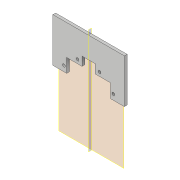
# Autodesk Inventor part: Hang Mount
Saved by Autodesk Inventor 2018 (Build 220112000, 112)
## iProperties
Created: 2018-01-17
Part Number: Hang Mount
Material: Generic
Document SubType Name: Modeling
Designer: dsayers
Density: 1 g/cm^3
Appearance: Default
Author: dsayers
Autodesk Inventor part; units mm, degrees
ref_plane "YZ Plane" through (0, 0, 0) normal (1, 0, 0) x (0, 1, 0)
ref_plane "XZ Plane" through (0, 0, 0) normal (0, 1, 0) x (-1, 0, 0)
ref_plane "XY Plane" through (0, 0, 0) normal (0, 0, 1) x (1, 0, 0)
ref_plane "Work Plane1" through (0, 0, 0) normal (0, 0, 1) x (1, 0, 0)
sketch "Sketch2" plane through (0, 0, 0) normal (0, 0, 1) x (1, 0, 0)
  line L0 (-69.85, 121.9708) -> (69.85, 121.9708) projected
  line L1 (-69.85, 33.0708) -> (-69.85, 121.9708) projected
  line L2 (69.85, 33.0708) -> (-69.85, 33.0708) projected
  line L3 (-50.8, 64.8208) -> (-50.8, 33.0708) projected
  line L4 (50.8, 64.8208) -> (-50.8, 64.8208) projected
  line L5 (50.8, 33.0708) -> (50.8, 64.8208) projected
  line L6 (69.85, 121.9708) -> (69.85, 33.0708) projected
  line L7 (-15.2718, 85.3756) -> (-15.2718, 64.8208) projected
  line L8 (15.24, 85.3756) -> (-15.2718, 85.3756) projected
  line L9 (15.24, 64.8208) -> (15.24, 85.3756) projected
  point P0 (0, 0)
extrude "Extrusion1" add sketch "Sketch2" along normal blind 6.35 contours L0 L6 L2 L5 L4 L9 L8 L7 L3 L1
sketch "Sketch3" plane through (0, 0, 6.35) normal (0, 0, 1) x (1, 0, 0)
  circle A0 centre (-57.15, 45.7708) radius 3.5662 projected
  circle A1 centre (-25.4, 73.7616) radius 2.4892 projected
  circle A2 centre (57.15, 45.7708) radius 3.9624 projected
  point P0 (0, 0)
  point P1 (25.4, 73.7616)
  point P2 (25.4, 73.7616)
  constraints: 4 coincident
hole "Hole1" at (25.4, 73.7616, 6.35) at (-57.15, 45.7708, 6.35) at (57.15, 45.7708, 6.35) at (-25.4, 73.7616, 6.35) direction (0, 0, -1) diameter 6.35 depth 25.4 tip angle 118
sketch "Sketch5" plane through (0, 0, 6.35) normal (0, 0, 1) x (1, 0, 0)
  line L0 (-69.85, 33.0708) -> (-50.8, 33.0708) projected
  line L1 (-69.85, 33.0708) -> (-82.55, 33.0708)
  line L2 (-82.55, 33.0708) -> (-82.55, 134.6708)
  line L3 (-82.55, 134.6708) -> (-69.85, 134.6708)
  line L4 (-69.85, 134.6708) -> (-69.85, 33.0708)
  line L5 (-82.55, 134.6708) -> (82.55, 134.6708)
  line L6 (82.55, 134.6708) -> (82.55, 121.9708)
  line L7 (82.55, 121.9708) -> (-82.55, 121.9708)
  line L8 (-82.55, 121.9708) -> (-82.55, 134.6708)
  line L9 (50.8, 33.0708) -> (69.85, 33.0708) projected
  line L10 (82.55, 121.9708) -> (69.85, 121.9708)
  line L11 (69.85, 121.9708) -> (69.85, 33.0708)
  line L12 (69.85, 33.0708) -> (82.55, 33.0708)
  line L13 (82.55, 33.0708) -> (82.55, 121.9708)
  point P0 (0, 0)
  dimension "d26" = 12.7
  dimension "d27" = 12.7
  dimension "d28" = 12.7
  constraints: 24 end point, 6 parallel, 3 horizontal, 3 perpendicular
  measures "d26" distance between parallel lines of L11 L13
  measures "d27" distance between parallel lines of L7 L5
  measures "d28" distance between parallel lines of L2 L4
extrude "Extrusion3" add sketch "Sketch5" against normal up to surface (6.35 mm away)
ref_plane "Work Plane2" through (0, 33.0708, 6.35) normal (-1, 0, 0) x (0, 0, 1)
equation "\"d1\" = d2"
equation "\"d2\" = 12.7"
body "Solid1"
